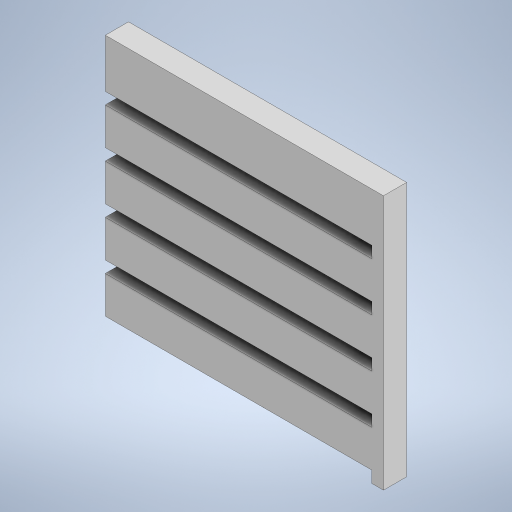
# Autodesk Inventor part: NewBackPlate
Saved by Autodesk Inventor 2024 (Build 280153000, 153)
## iProperties
Created: 2023-10-24
Part Number: NewBackPlate
Material: Generic
Document SubType Name: Modeling
Designer: flynf
Density: 1 g/cm^3
Appearance: Default
Author: flynf
Autodesk Inventor part; units mm, degrees
ref_plane "YZ Plane" through (0, 0, 0) normal (1, 0, 0) x (0, 1, 0)
ref_plane "XZ Plane" through (0, 0, 0) normal (0, 1, 0) x (-1, 0, 0)
ref_plane "XY Plane" through (0, 0, 0) normal (0, 0, 1) x (1, 0, 0)
sketch "Sketch1" plane through (0, 0, 0) normal (0, 0, 1) x (1, 0, 0)
  line L0 (0, 0) -> (279.4, 0)
  line L1 (279.4, 0) -> (279.4, 279.4)
  line L2 (279.4, 279.4) -> (0, 279.4)
  line L3 (0, 279.4) -> (0, 0)
  dimension "d0" = 279.4
  dimension "d1" = 279.4
  constraints: 8 end point, 2 parallel, 1 horizontal, 1 perpendicular
  measures "d0" distance of L0.start L0.end
  measures "d1" distance of L0.end L1.end
extrude "Extrusion1" add sketch "Sketch1" along normal blind 25.4
sketch "Sketch2" plane through (0, 0, 25.4) normal (0, 0, 1) x (1, 0, 0)
  line L0 (0, 279.4) -> (0, 0) projected
  line L1 (0, 213.36) -> (266.7, 213.36)
  line L2 (266.7, 213.36) -> (266.7, 226.06)
  line L3 (266.7, 226.06) -> (0, 226.06)
  line L4 (0, 226.06) -> (0, 213.36)
  line L5 (279.4, 279.4) -> (0, 279.4) projected
  line L6 (0, 106.68) -> (266.7, 106.68)
  line L7 (266.7, 106.68) -> (266.7, 119.38)
  line L8 (266.7, 119.38) -> (0, 119.38)
  line L9 (0, 119.38) -> (0, 106.68)
  line L10 (0, 0) -> (266.7, 0)
  line L11 (266.7, 0) -> (266.7, 12.7)
  line L12 (266.7, 12.7) -> (0, 12.7)
  line L13 (0, 12.7) -> (0, 0)
  line L14 (0, 53.34) -> (266.7, 53.34)
  line L15 (266.7, 53.34) -> (266.7, 66.04)
  line L16 (266.7, 66.04) -> (0, 66.04)
  line L17 (0, 66.04) -> (0, 53.34)
  line L18 (0, 160.02) -> (266.7, 160.02)
  line L19 (266.7, 160.02) -> (266.7, 172.72)
  line L20 (266.7, 172.72) -> (0, 172.72)
  line L21 (0, 172.72) -> (0, 160.02)
  point P0 (0, 226.06)
  point P1 (0, 172.72)
  point P2 (0, 119.38)
  point P3 (0, 66.04)
  point P4 (0, 12.7)
  dimension "d4" = 266.7
  dimension "d5" = 12.7
  dimension "d6" = 53.34
  dimension "d7" = 266.7
  dimension "d8" = 0
  dimension "d9" = 0
  dimension "d10" = 0
  dimension "d11" = 0
  dimension "d12" = 266.7
  dimension "d13" = 266.7
  dimension "d14" = 266.7
  dimension "d15" = 12.7
  dimension "d16" = 40.64
  dimension "d17" = 12.7
  dimension "d18" = 40.64
  dimension "d19" = 12.7
  dimension "d20" = 12.7
  dimension "d21" = 40.64
  dimension "d22" = 40.64
  constraints: 40 end point, 10 parallel, 5 horizontal, 5 perpendicular, 1 point on line
  measures "d4" distance of L2.end L3.end
  measures "d5" distance of L1.end L2.end
  measures "d6" distance between parallel lines of L5 L3
  measures "d7" distance of L19.end L20.end
  measures "d8" distance between parallel lines of L0 L21
  measures "d9" distance between parallel lines of L0 L9
  measures "d10" distance between parallel lines of L0 L17
  measures "d11" distance between parallel lines of L0 L13
  measures "d12" distance of L7.end L8.end
  measures "d13" distance of L15.end L16.end
  measures "d14" distance of L11.end L12.end
  measures "d15" distance between parallel lines of L20 L18
  measures "d16" distance between parallel lines of L1 L20
  measures "d17" distance between parallel lines of L6 L8
  measures "d18" distance between parallel lines of L18 L8
  measures "d19" distance between parallel lines of L16 L14
  measures "d20" distance between parallel lines of L12 L10
  measures "d21" distance between parallel lines of L6 L16
  measures "d22" distance between parallel lines of L14 L12
extrude "Extrusion2" cut sketch "Sketch2" against normal blind 12.7
sketch "Sketch3" plane through (0, 0, 0) normal (-1, 0, 0) x (0, 0, 1)
  line L0 (0, 279.4) -> (0, 0) projected
  line L1 (12.7, 226.06) -> (25.4, 226.06) projected
  line L2 (0, 279.4) -> (25.4, 279.4)
  line L3 (25.4, 279.4) -> (25.4, 226.06)
  line L4 (25.4, 226.06) -> (0, 226.06)
  line L5 (0, 226.06) -> (0, 279.4)
  line L6 (25.4, 213.36) -> (12.7, 213.36) projected
  line L7 (25.4, 213.36) -> (0, 213.36)
  line L8 (0, 213.36) -> (0, 172.72)
  line L9 (0, 172.72) -> (25.4, 172.72)
  line L10 (25.4, 172.72) -> (25.4, 213.36)
  line L11 (25.4, 160.02) -> (25.4, 119.38) projected
  line L12 (25.4, 160.02) -> (0, 160.02)
  line L13 (0, 160.02) -> (0, 119.38)
  line L14 (0, 119.38) -> (25.4, 119.38)
  line L15 (25.4, 119.38) -> (25.4, 160.02)
  line L16 (25.4, 106.68) -> (25.4, 66.04) projected
  line L17 (25.4, 106.68) -> (0, 106.68)
  line L18 (0, 106.68) -> (0, 66.04)
  line L19 (0, 66.04) -> (25.4, 66.04)
  line L20 (25.4, 66.04) -> (25.4, 106.68)
  line L21 (25.4, 53.34) -> (12.7, 53.34) projected
  line L22 (25.4, 53.34) -> (0, 53.34)
  line L23 (0, 53.34) -> (0, 12.7)
  line L24 (0, 12.7) -> (25.4, 12.7)
  line L25 (25.4, 12.7) -> (25.4, 53.34)
  dimension "d25" = 40.64
  dimension "d26" = 25.4
  dimension "d27" = 40.64
  dimension "d28" = 25.4
  dimension "d29" = 40.64
  dimension "d30" = 25.4
  dimension "d31" = 40.64
  constraints: 40 end point, 10 parallel, 5 horizontal, 5 perpendicular, 1 point on line
  measures "d25" distance of L8.end L7.end
  measures "d26" distance of L14.end L13.end
  measures "d27" distance of L13.end L12.end
  measures "d28" distance of L19.end L18.end
  measures "d29" distance of L18.end L17.end
  measures "d30" distance of L24.end L23.end
  measures "d31" distance of L23.end L22.end
extrude "Extrusion3" add sketch "Sketch3" along normal blind 25.4
body "Solid1"
